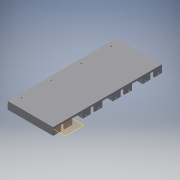
# Autodesk Inventor part: Syring Pump Holder
Saved by Autodesk Inventor 2018.1 (Build 221171000, 171)
## iProperties
Created: 2024-06-08
Part Number: Syring Pump Holder
Material: Generic
Document SubType Name: Modeling
Designer: Enrico
Density: 1 g/cm^3
Appearance: Default
Author: Enrico
Autodesk Inventor part; units mm, degrees
ref_plane "YZ Plane" through (0, 0, 0) normal (1, 0, 0) x (0, 1, 0)
ref_plane "XZ Plane" through (0, 0, 0) normal (0, 1, 0) x (-1, 0, 0)
ref_plane "XY Plane" through (0, 0, 0) normal (0, 0, 1) x (1, 0, 0)
ref_plane "Work Plane1" through (0, 0, 0) normal (0, 0, 1) x (1, 0, 0)
sketch "Sketch1" plane through (0, 0, 0) normal (0, 0, 1) x (1, 0, 0)
  line L0 (57.1, 22.5) -> (57.1, -22.5) construction
  line L1 (57.1, 22.5) -> (-58.1, 22.5) construction
  line L2 (-58.1, 22.5) -> (-58.1, -22.5) construction
  line L3 (-58.1, -22.5) -> (57.1, -22.5) construction
  arc A0 (47.6, -19.5) -> (49.6, -17.5) centre (47.6, -17.5) ccw construction
  line L4 (47.6, -19.5) -> (-47.1, -19.5) construction
  line L5 (-47.1, -19.5) -> (-47.1, -6.5) construction
  arc A1 (-47.1, -6.5) -> (-49.1, -4.5) centre (-49.1, -6.5) ccw construction
  line L6 (-49.1, -4.5) -> (-52.1, -4.5) construction
  arc A2 (-54.1, -2.5) -> (-52.1, -4.5) centre (-52.1, -2.5) ccw construction
  line L7 (-54.1, -2.5) -> (-54.1, 2.5) construction
  arc A3 (-52.1, 4.5) -> (-54.1, 2.5) centre (-52.1, 2.5) ccw construction
  line L8 (-52.1, 4.5) -> (-49.1, 4.5) construction
  arc A4 (-49.1, 4.5) -> (-47.1, 6.5) centre (-49.1, 6.5) ccw construction
  line L9 (-47.1, 6.5) -> (-47.1, 19.5) construction
  line L10 (-47.1, 19.5) -> (47.6, 19.5) construction
  arc A5 (49.6, 17.5) -> (47.6, 19.5) centre (47.6, 17.5) ccw construction
  line L11 (49.6, 17.5) -> (49.6, 9.5) construction
  arc A6 (47.6, 7.5) -> (49.6, 9.5) centre (47.6, 9.5) ccw construction
  line L12 (47.6, 7.5) -> (42.1, 7.5) construction
  arc A7 (42.1, 7.5) -> (40.1, 5.5) centre (42.1, 5.5) ccw construction
  line L13 (40.1, 5.5) -> (40.1, -5.5) construction
  arc A8 (40.1, -5.5) -> (42.1, -7.5) centre (42.1, -5.5) ccw construction
  line L14 (42.1, -7.5) -> (47.6, -7.5) construction
  arc A9 (49.6, -9.5) -> (47.6, -7.5) centre (47.6, -9.5) ccw construction
  line L15 (49.6, -9.5) -> (49.6, -17.5) construction
  line L16 (57.1, 102.5) -> (57.1, 57.5) construction
  line L17 (57.1, 102.5) -> (-58.1, 102.5) construction
  line L18 (-58.1, 102.5) -> (-58.1, 57.5) construction
  line L19 (-58.1, 57.5) -> (57.1, 57.5) construction
  arc A10 (47.6, 60.5) -> (49.6, 62.5) centre (47.6, 62.5) ccw construction
  line L20 (47.6, 60.5) -> (-47.1, 60.5) construction
  line L21 (-47.1, 60.5) -> (-47.1, 73.5) construction
  arc A11 (-47.1, 73.5) -> (-49.1, 75.5) centre (-49.1, 73.5) ccw construction
  line L22 (-49.1, 75.5) -> (-52.1, 75.5) construction
  arc A12 (-54.1, 77.5) -> (-52.1, 75.5) centre (-52.1, 77.5) ccw construction
  line L23 (-54.1, 77.5) -> (-54.1, 82.5) construction
  arc A13 (-52.1, 84.5) -> (-54.1, 82.5) centre (-52.1, 82.5) ccw construction
  line L24 (-52.1, 84.5) -> (-49.1, 84.5) construction
  arc A14 (-49.1, 84.5) -> (-47.1, 86.5) centre (-49.1, 86.5) ccw construction
  line L25 (-47.1, 86.5) -> (-47.1, 99.5) construction
  line L26 (-47.1, 99.5) -> (47.6, 99.5) construction
  arc A15 (49.6, 97.5) -> (47.6, 99.5) centre (47.6, 97.5) ccw construction
  line L27 (49.6, 97.5) -> (49.6, 89.5) construction
  arc A16 (47.6, 87.5) -> (49.6, 89.5) centre (47.6, 89.5) ccw construction
  line L28 (47.6, 87.5) -> (42.1, 87.5) construction
  arc A17 (42.1, 87.5) -> (40.1, 85.5) centre (42.1, 85.5) ccw construction
  line L29 (40.1, 85.5) -> (40.1, 74.5) construction
  arc A18 (40.1, 74.5) -> (42.1, 72.5) centre (42.1, 74.5) ccw construction
  line L30 (42.1, 72.5) -> (47.6, 72.5) construction
  arc A19 (49.6, 70.5) -> (47.6, 72.5) centre (47.6, 70.5) ccw construction
  line L31 (49.6, 70.5) -> (49.6, 62.5) construction
  line L32 (57.1, 182.5) -> (57.1, 137.5) construction
  line L33 (57.1, 182.5) -> (-58.1, 182.5) construction
  line L34 (-58.1, 182.5) -> (-58.1, 137.5) construction
  line L35 (-58.1, 137.5) -> (57.1, 137.5) construction
  arc A20 (47.6, 140.5) -> (49.6, 142.5) centre (47.6, 142.5) ccw construction
  line L36 (47.6, 140.5) -> (-47.1, 140.5) construction
  line L37 (-47.1, 140.5) -> (-47.1, 153.5) construction
  arc A21 (-47.1, 153.5) -> (-49.1, 155.5) centre (-49.1, 153.5) ccw construction
  line L38 (-49.1, 155.5) -> (-52.1, 155.5) construction
  arc A22 (-54.1, 157.5) -> (-52.1, 155.5) centre (-52.1, 157.5) ccw construction
  line L39 (-54.1, 157.5) -> (-54.1, 162.5) construction
  arc A23 (-52.1, 164.5) -> (-54.1, 162.5) centre (-52.1, 162.5) ccw construction
  line L40 (-52.1, 164.5) -> (-49.1, 164.5) construction
  arc A24 (-49.1, 164.5) -> (-47.1, 166.5) centre (-49.1, 166.5) ccw construction
  line L41 (-47.1, 166.5) -> (-47.1, 179.5) construction
  line L42 (-47.1, 179.5) -> (47.6, 179.5) construction
  arc A25 (49.6, 177.5) -> (47.6, 179.5) centre (47.6, 177.5) ccw construction
  line L43 (49.6, 177.5) -> (49.6, 169.5) construction
  arc A26 (47.6, 167.5) -> (49.6, 169.5) centre (47.6, 169.5) ccw construction
  line L44 (47.6, 167.5) -> (42.1, 167.5) construction
  arc A27 (42.1, 167.5) -> (40.1, 165.5) centre (42.1, 165.5) ccw construction
  line L45 (40.1, 165.5) -> (40.1, 154.5) construction
  arc A28 (40.1, 154.5) -> (42.1, 152.5) centre (42.1, 154.5) ccw construction
  line L46 (42.1, 152.5) -> (47.6, 152.5) construction
  arc A29 (49.6, 150.5) -> (47.6, 152.5) centre (47.6, 150.5) ccw construction
  line L47 (49.6, 150.5) -> (49.6, 142.5) construction
  line L48 (57.1, 262.5) -> (57.1, 217.5) construction
  line L49 (57.1, 262.5) -> (-58.1, 262.5) construction
  line L50 (-58.1, 262.5) -> (-58.1, 217.5) construction
  line L51 (-58.1, 217.5) -> (57.1, 217.5) construction
  arc A30 (47.6, 220.5) -> (49.6, 222.5) centre (47.6, 222.5) ccw construction
  line L52 (47.6, 220.5) -> (-47.1, 220.5) construction
  line L53 (-47.1, 220.5) -> (-47.1, 233.5) construction
  arc A31 (-47.1, 233.5) -> (-49.1, 235.5) centre (-49.1, 233.5) ccw construction
  line L54 (-49.1, 235.5) -> (-52.1, 235.5) construction
  arc A32 (-54.1, 237.5) -> (-52.1, 235.5) centre (-52.1, 237.5) ccw construction
  line L55 (-54.1, 237.5) -> (-54.1, 242.5) construction
  arc A33 (-52.1, 244.5) -> (-54.1, 242.5) centre (-52.1, 242.5) ccw construction
  line L56 (-52.1, 244.5) -> (-49.1, 244.5) construction
  arc A34 (-49.1, 244.5) -> (-47.1, 246.5) centre (-49.1, 246.5) ccw construction
  line L57 (-47.1, 246.5) -> (-47.1, 259.5) construction
  line L58 (-47.1, 259.5) -> (47.6, 259.5) construction
  arc A35 (49.6, 257.5) -> (47.6, 259.5) centre (47.6, 257.5) ccw construction
  line L59 (49.6, 257.5) -> (49.6, 249.5) construction
  arc A36 (47.6, 247.5) -> (49.6, 249.5) centre (47.6, 249.5) ccw construction
  line L60 (47.6, 247.5) -> (42.1, 247.5) construction
  arc A37 (42.1, 247.5) -> (40.1, 245.5) centre (42.1, 245.5) ccw construction
  line L61 (40.1, 245.5) -> (40.1, 234.5) construction
  arc A38 (40.1, 234.5) -> (42.1, 232.5) centre (42.1, 234.5) ccw construction
  line L62 (42.1, 232.5) -> (47.6, 232.5) construction
  arc A39 (49.6, 230.5) -> (47.6, 232.5) centre (47.6, 230.5) ccw construction
  line L63 (49.6, 230.5) -> (49.6, 222.5) construction
  circle A40 centre (-49.9, 240) radius 1.5 projected
  arc A41 (-26, 167) -> (-26, 153) centre (-26, 160) ccw construction
  line L64 (-26, 167) -> (26, 167) construction
  arc A42 (26, 153) -> (26, 167) centre (26, 160) ccw construction
  line L65 (26, 153) -> (-26, 153) construction
  circle A43 centre (44.1, 147) radius 1.5 construction
  circle A44 centre (44.1, 173) radius 1.5 construction
  circle A45 centre (-49.9, 160) radius 1.5 projected
  line L66 (47.6, 140.5) -> (-47.1, 140.5) construction
  arc A46 (47.6, 140.5) -> (49.6, 142.5) centre (47.6, 142.5) ccw construction
  line L67 (49.6, 150.5) -> (49.6, 142.5) construction
  arc A47 (49.6, 150.5) -> (47.6, 152.5) centre (47.6, 150.5) ccw construction
  line L68 (42.1, 152.5) -> (47.6, 152.5) construction
  arc A48 (40.1, 154.5) -> (42.1, 152.5) centre (42.1, 154.5) ccw construction
  line L69 (40.1, 165.5) -> (40.1, 154.5) construction
  arc A49 (42.1, 167.5) -> (40.1, 165.5) centre (42.1, 165.5) ccw construction
  line L70 (47.6, 167.5) -> (42.1, 167.5) construction
  arc A50 (47.6, 167.5) -> (49.6, 169.5) centre (47.6, 169.5) ccw construction
  line L71 (49.6, 177.5) -> (49.6, 169.5) construction
  arc A51 (49.6, 177.5) -> (47.6, 179.5) centre (47.6, 177.5) ccw construction
  line L72 (-47.1, 179.5) -> (47.6, 179.5) construction
  line L73 (-47.1, 166.5) -> (-47.1, 179.5) construction
  arc A52 (-49.1, 164.5) -> (-47.1, 166.5) centre (-49.1, 166.5) ccw construction
  line L74 (-52.1, 164.5) -> (-49.1, 164.5) construction
  arc A53 (-52.1, 164.5) -> (-54.1, 162.5) centre (-52.1, 162.5) ccw construction
  line L75 (-54.1, 157.5) -> (-54.1, 162.5) construction
  arc A54 (-54.1, 157.5) -> (-52.1, 155.5) centre (-52.1, 157.5) ccw construction
  line L76 (-49.1, 155.5) -> (-52.1, 155.5) construction
  arc A55 (-47.1, 153.5) -> (-49.1, 155.5) centre (-49.1, 153.5) ccw construction
  line L77 (-47.1, 140.5) -> (-47.1, 153.5) construction
  arc A56 (-26, 87) -> (-26, 73) centre (-26, 80) ccw construction
  line L78 (-26, 87) -> (26, 87) construction
  arc A57 (26, 73) -> (26, 87) centre (26, 80) ccw construction
  line L79 (26, 73) -> (-26, 73) construction
  circle A58 centre (44.1, 67) radius 1.5 construction
  circle A59 centre (44.1, 93) radius 1.5 construction
  circle A60 centre (-49.9, 80) radius 1.5 projected
  line L80 (47.6, 60.5) -> (-47.1, 60.5) construction
  arc A61 (47.6, 60.5) -> (49.6, 62.5) centre (47.6, 62.5) ccw construction
  line L81 (49.6, 70.5) -> (49.6, 62.5) construction
  arc A62 (49.6, 70.5) -> (47.6, 72.5) centre (47.6, 70.5) ccw construction
  line L82 (42.1, 72.5) -> (47.6, 72.5) construction
  arc A63 (40.1, 74.5) -> (42.1, 72.5) centre (42.1, 74.5) ccw construction
  line L83 (40.1, 85.5) -> (40.1, 74.5) construction
  arc A64 (42.1, 87.5) -> (40.1, 85.5) centre (42.1, 85.5) ccw construction
  line L84 (47.6, 87.5) -> (42.1, 87.5) construction
  arc A65 (47.6, 87.5) -> (49.6, 89.5) centre (47.6, 89.5) ccw construction
  line L85 (49.6, 97.5) -> (49.6, 89.5) construction
  arc A66 (49.6, 97.5) -> (47.6, 99.5) centre (47.6, 97.5) ccw construction
  line L86 (-47.1, 99.5) -> (47.6, 99.5) construction
  line L87 (-47.1, 86.5) -> (-47.1, 99.5) construction
  arc A67 (-49.1, 84.5) -> (-47.1, 86.5) centre (-49.1, 86.5) ccw construction
  line L88 (-52.1, 84.5) -> (-49.1, 84.5) construction
  arc A68 (-52.1, 84.5) -> (-54.1, 82.5) centre (-52.1, 82.5) ccw construction
  line L89 (-54.1, 77.5) -> (-54.1, 82.5) construction
  arc A69 (-54.1, 77.5) -> (-52.1, 75.5) centre (-52.1, 77.5) ccw construction
  line L90 (-49.1, 75.5) -> (-52.1, 75.5) construction
  arc A70 (-47.1, 73.5) -> (-49.1, 75.5) centre (-49.1, 73.5) ccw construction
  line L91 (-47.1, 60.5) -> (-47.1, 73.5) construction
  arc A71 (-26, 7) -> (-26, -7) centre (-26, 0) ccw construction
  line L92 (-26, 7) -> (26, 7) construction
  arc A72 (26, -7) -> (26, 7) centre (26, 0) ccw construction
  line L93 (26, -7) -> (-26, -7) construction
  circle A73 centre (44.1, -13) radius 1.5 construction
  circle A74 centre (44.1, 13) radius 1.5 construction
  circle A75 centre (-49.9, 0) radius 1.5 projected
  line L94 (47.6, -19.5) -> (-47.1, -19.5) construction
  arc A76 (47.6, -19.5) -> (49.6, -17.5) centre (47.6, -17.5) ccw construction
  line L95 (49.6, -9.5) -> (49.6, -17.5) construction
  arc A77 (49.6, -9.5) -> (47.6, -7.5) centre (47.6, -9.5) ccw construction
  line L96 (42.1, -7.5) -> (47.6, -7.5) construction
  arc A78 (40.1, -5.5) -> (42.1, -7.5) centre (42.1, -5.5) ccw construction
  line L97 (40.1, 5.5) -> (40.1, -5.5) construction
  arc A79 (42.1, 7.5) -> (40.1, 5.5) centre (42.1, 5.5) ccw construction
  line L98 (47.6, 7.5) -> (42.1, 7.5) construction
  arc A80 (47.6, 7.5) -> (49.6, 9.5) centre (47.6, 9.5) ccw construction
  line L99 (49.6, 17.5) -> (49.6, 9.5) construction
  arc A81 (49.6, 17.5) -> (47.6, 19.5) centre (47.6, 17.5) ccw construction
  line L100 (-47.1, 19.5) -> (47.6, 19.5) construction
  line L101 (-47.1, 6.5) -> (-47.1, 19.5) construction
  arc A82 (-49.1, 4.5) -> (-47.1, 6.5) centre (-49.1, 6.5) ccw construction
  line L102 (-52.1, 4.5) -> (-49.1, 4.5) construction
  arc A83 (-52.1, 4.5) -> (-54.1, 2.5) centre (-52.1, 2.5) ccw construction
  line L103 (-54.1, -2.5) -> (-54.1, 2.5) construction
  arc A84 (-54.1, -2.5) -> (-52.1, -4.5) centre (-52.1, -2.5) ccw construction
  line L104 (-49.1, -4.5) -> (-52.1, -4.5) construction
  arc A85 (-47.1, -6.5) -> (-49.1, -4.5) centre (-49.1, -6.5) ccw construction
  line L105 (-47.1, -19.5) -> (-47.1, -6.5) construction
  arc A86 (-26, 247) -> (-26, 233) centre (-26, 240) ccw construction
  line L106 (-26, 247) -> (26, 247) construction
  arc A87 (26, 233) -> (26, 247) centre (26, 240) ccw construction
  line L107 (26, 233) -> (-26, 233) construction
  circle A88 centre (44.1, 227) radius 1.5 construction
  circle A89 centre (44.1, 253) radius 1.5 construction
  circle A90 centre (-49.9, 240) radius 1.5 construction
  line L108 (47.6, 220.5) -> (-47.1, 220.5) construction
  arc A91 (47.6, 220.5) -> (49.6, 222.5) centre (47.6, 222.5) ccw construction
  line L109 (49.6, 230.5) -> (49.6, 222.5) construction
  arc A92 (49.6, 230.5) -> (47.6, 232.5) centre (47.6, 230.5) ccw construction
  line L110 (42.1, 232.5) -> (47.6, 232.5) construction
  arc A93 (40.1, 234.5) -> (42.1, 232.5) centre (42.1, 234.5) ccw construction
  line L111 (40.1, 245.5) -> (40.1, 234.5) construction
  arc A94 (42.1, 247.5) -> (40.1, 245.5) centre (42.1, 245.5) ccw construction
  line L112 (47.6, 247.5) -> (42.1, 247.5) construction
  arc A95 (47.6, 247.5) -> (49.6, 249.5) centre (47.6, 249.5) ccw construction
  line L113 (49.6, 257.5) -> (49.6, 249.5) construction
  arc A96 (49.6, 257.5) -> (47.6, 259.5) centre (47.6, 257.5) ccw construction
  line L114 (-47.1, 259.5) -> (47.6, 259.5) construction
  line L115 (-47.1, 246.5) -> (-47.1, 259.5) construction
  arc A97 (-49.1, 244.5) -> (-47.1, 246.5) centre (-49.1, 246.5) ccw construction
  line L116 (-52.1, 244.5) -> (-49.1, 244.5) construction
  arc A98 (-52.1, 244.5) -> (-54.1, 242.5) centre (-52.1, 242.5) ccw construction
  line L117 (-54.1, 237.5) -> (-54.1, 242.5) construction
  arc A99 (-54.1, 237.5) -> (-52.1, 235.5) centre (-52.1, 237.5) ccw construction
  line L118 (-49.1, 235.5) -> (-52.1, 235.5) construction
  arc A100 (-47.1, 233.5) -> (-49.1, 235.5) centre (-49.1, 233.5) ccw construction
  line L119 (-47.1, 220.5) -> (-47.1, 233.5) construction
  line L120 (60.4, 265.8) -> (-61.4, 265.8)
  line L121 (-61.4, 265.8) -> (-61.4, -25.8)
  line L122 (-61.4, -25.8) -> (60.4, -25.8)
  line L123 (60.4, -25.8) -> (60.4, 265.8)
  point P0 (0, 0)
  dimension "d0" = 3.3
  dimension "d1" = 3.3
  dimension "d2" = 3.3
  dimension "d3" = 3.3
  constraints: 8 end point, 2 parallel, 1 horizontal, 1 perpendicular
  measures "d0" distance between parallel lines of L49 L120
  measures "d1" distance between parallel lines of L48 L123
  measures "d2" distance between parallel lines of L50 L121
  measures "d3" distance between parallel lines of L3 L122
extrude "Extrusion1" add sketch "Sketch1" along normal blind 5
sketch "Sketch2" plane through (0, 0, 0) normal (0, 0, -1) x (-1, 0, 0)
  line L0 (-57.1, -22.5) -> (-57.1, 22.5) construction
  line L1 (-57.1, -22.5) -> (58.1, -22.5) construction
  line L2 (58.1, -22.5) -> (58.1, 22.5) construction
  line L3 (58.1, 22.5) -> (-57.1, 22.5) construction
  circle A0 centre (-55.1, -16.5) radius 1.5 construction
  circle A1 centre (-55.1, 16.5) radius 1.5 construction
  line L4 (-57.1, 57.5) -> (-57.1, 102.5) construction
  line L5 (-57.1, 57.5) -> (58.1, 57.5) construction
  line L6 (58.1, 57.5) -> (58.1, 102.5) construction
  line L7 (58.1, 102.5) -> (-57.1, 102.5) construction
  circle A2 centre (-55.1, 63.5) radius 1.5 construction
  circle A3 centre (-55.1, 96.5) radius 1.5 construction
  line L8 (-57.1, 137.5) -> (-57.1, 182.5) construction
  line L9 (-57.1, 137.5) -> (58.1, 137.5) construction
  line L10 (58.1, 137.5) -> (58.1, 182.5) construction
  line L11 (58.1, 182.5) -> (-57.1, 182.5) construction
  circle A4 centre (-55.1, 143.5) radius 1.5 construction
  circle A5 centre (-55.1, 176.5) radius 1.5 construction
  line L12 (-57.1, 217.5) -> (-57.1, 262.5) construction
  line L13 (-57.1, 217.5) -> (58.1, 217.5) construction
  line L14 (58.1, 217.5) -> (58.1, 262.5) construction
  line L15 (58.1, 262.5) -> (-57.1, 262.5) construction
  circle A6 centre (-55.1, 223.5) radius 1.5 construction
  circle A7 centre (-55.1, 256.5) radius 1.5 construction
  line L16 (58.4, 217.2) -> (-57.4, 217.2)
  line L17 (-57.4, 217.2) -> (-57.4, 262.8)
  line L18 (-57.4, 262.8) -> (58.4, 262.8)
  line L19 (58.4, 262.8) -> (58.4, 217.2)
  line L20 (58.4, 137.2) -> (-57.4, 137.2)
  line L21 (-57.4, 137.2) -> (-57.4, 182.8)
  line L22 (-57.4, 182.8) -> (58.4, 182.8)
  line L23 (58.4, 182.8) -> (58.4, 137.2)
  line L24 (58.4, 57.2) -> (-57.4, 57.2)
  line L25 (-57.4, 57.2) -> (-57.4, 102.8)
  line L26 (-57.4, 102.8) -> (58.4, 102.8)
  line L27 (58.4, 102.8) -> (58.4, 57.2)
  line L28 (58.4, -22.8) -> (-57.4, -22.8)
  line L29 (-57.4, -22.8) -> (-57.4, 22.8)
  line L30 (-57.4, 22.8) -> (58.4, 22.8)
  line L31 (58.4, 22.8) -> (58.4, -22.8)
  line L32 (-60.4, -25.8) -> (61.4, -25.8)
  line L33 (61.4, -25.8) -> (61.4, 25.8)
  line L34 (61.4, 25.8) -> (-60.4, 25.8)
  line L35 (-60.4, 25.8) -> (-60.4, -25.8)
  line L36 (-60.4, 54.2) -> (61.4, 54.2)
  line L37 (61.4, 54.2) -> (61.4, 105.8)
  line L38 (61.4, 105.8) -> (-60.4, 105.8)
  line L39 (-60.4, 105.8) -> (-60.4, 54.2)
  line L40 (-60.4, 134.2) -> (61.4, 134.2)
  line L41 (61.4, 134.2) -> (61.4, 185.8)
  line L42 (61.4, 185.8) -> (-60.4, 185.8)
  line L43 (-60.4, 185.8) -> (-60.4, 134.2)
  line L44 (-60.4, 214.2) -> (61.4, 214.2)
  line L45 (61.4, 214.2) -> (61.4, 265.8)
  line L46 (61.4, 265.8) -> (-60.4, 265.8)
  line L47 (-60.4, 265.8) -> (-60.4, 214.2)
  line L48 (-85.2, 244.5) -> (-85.2, 235.5) projected
  line L49 (-58.1, 244.5) -> (-85.2, 244.5) projected
  line L50 (-58.1, 235.5) -> (-58.1, 244.5) projected
  line L51 (-85.2, 235.5) -> (-58.1, 235.5) projected
  line L52 (-85.2, 164.5) -> (-85.2, 155.5) projected
  line L53 (-58.1, 164.5) -> (-85.2, 164.5) projected
  line L54 (-58.1, 155.5) -> (-58.1, 164.5) projected
  line L55 (-85.2, 155.5) -> (-58.1, 155.5) projected
  line L56 (-85.2, 84.5) -> (-85.2, 75.5) projected
  line L57 (-58.1, 84.5) -> (-85.2, 84.5) projected
  line L58 (-58.1, 75.5) -> (-58.1, 84.5) projected
  line L59 (-85.2, 75.5) -> (-58.1, 75.5) projected
  line L60 (-85.2, 4.5) -> (-85.2, -4.5) projected
  line L61 (-58.1, 4.5) -> (-85.2, 4.5) projected
  line L62 (-58.1, -4.5) -> (-58.1, 4.5) projected
  line L63 (-85.2, -4.5) -> (-58.1, -4.5) projected
  line L64 (-85.5, 244.8) -> (-85.5, 235.2)
  line L65 (-85.5, 235.2) -> (-57.8, 235.2)
  line L66 (-57.8, 235.2) -> (-57.8, 244.8)
  line L67 (-57.8, 244.8) -> (-85.5, 244.8)
  line L68 (-85.5, 164.8) -> (-85.5, 155.2)
  line L69 (-85.5, 155.2) -> (-57.8, 155.2)
  line L70 (-57.8, 155.2) -> (-57.8, 164.8)
  line L71 (-57.8, 164.8) -> (-85.5, 164.8)
  line L72 (-85.5, 84.8) -> (-85.5, 75.2)
  line L73 (-85.5, 75.2) -> (-57.8, 75.2)
  line L74 (-57.8, 75.2) -> (-57.8, 84.8)
  line L75 (-57.8, 84.8) -> (-85.5, 84.8)
  line L76 (-85.5, 4.8) -> (-85.5, -4.8)
  line L77 (-85.5, -4.8) -> (-57.8, -4.8)
  line L78 (-57.8, -4.8) -> (-57.8, 4.8)
  line L79 (-57.8, 4.8) -> (-85.5, 4.8) construction
  line L80 (-57.4, 4.8) -> (-60.4, 4.8)
  line L81 (-57.4, -4.8) -> (-60.4, -4.8)
  line L82 (-57.4, 84.8) -> (-60.4, 84.8)
  line L83 (-57.4, 75.2) -> (-60.4, 75.2)
  line L84 (-57.4, 164.8) -> (-60.4, 164.8)
  line L85 (-57.4, 155.2) -> (-60.4, 155.2)
  line L86 (-57.4, 244.8) -> (-60.4, 244.8)
  line L87 (-57.4, 235.2) -> (-60.4, 235.2)
  line L88 (-57.4, 244.8) -> (-60.4, 244.8)
  line L89 (-60.4, 244.8) -> (-60.4, 235.2)
  line L90 (-60.4, 235.2) -> (-57.4, 235.2)
  line L91 (-57.4, 235.2) -> (-57.4, 244.8)
  line L92 (-57.4, 164.8) -> (-60.4, 164.8)
  line L93 (-60.4, 164.8) -> (-60.4, 155.2)
  line L94 (-60.4, 155.2) -> (-57.4, 155.2)
  line L95 (-57.4, 155.2) -> (-57.4, 164.8)
  line L96 (-57.4, 84.8) -> (-60.4, 84.8)
  line L97 (-60.4, 84.8) -> (-60.4, 75.2)
  line L98 (-60.4, 75.2) -> (-57.4, 75.2)
  line L99 (-57.4, 75.2) -> (-57.4, 84.8)
  point P0 (0, 0)
  dimension "d6" = 0.3
  dimension "d7" = 0.3
  dimension "d8" = 0.3
  dimension "d9" = 0.3
  dimension "d10" = 3
  dimension "d11" = 3
  dimension "d12" = 3
  dimension "d13" = 3
  dimension "d14" = 0.3
  dimension "d15" = 0.3
  dimension "d16" = 0.3
  dimension "d17" = 0.3
  dimension "d20" = 80
  constraints: 136 end point, 6 parallel, 6 point on line, 3 horizontal, 3 perpendicular, 2 collinear, 1 vertical, 54 other
  measures "d6" distance between parallel lines of L13 L16
  measures "d7" distance between parallel lines of L9 L20
  measures "d8" distance between parallel lines of L5 L24
  measures "d9" distance between parallel lines of L1 L28
  measures "d10" distance between parallel lines of L28 L32
  measures "d11" distance between parallel lines of L24 L36
  measures "d12" distance between parallel lines of L20 L40
  measures "d13" distance between parallel lines of L16 L44
  measures "d14" distance between parallel lines of L49 L67
  measures "d15" distance between parallel lines of L53 L71
  measures "d16" distance between parallel lines of L57 L75
  measures "d17" distance between parallel lines of L61 L79
  measures "d20" distance of L80.start L82.start
extrude "Extrusion2" add sketch "Sketch2" along normal blind 15 contours L19 L18 L17 L86 L67 L47 L46 L45 L44 L65 L87 L16 | L23 L22 L21 L84 L71 L43 L42 L41 L40 L69 L85 L20 | L27 L26 L25 L82 L75 L39 L38 L37 L36 L73 L83 L24 | L31 L30 L29 L80 L35 L34 L33 L32 L77 L81 L28
sketch "Sketch3" plane through (60.4, -25.8, 5) normal (1, 0, 0) x (0, 0, -1)
  circle A0 centre (16.1, 8.55) radius 1.5 construction
  circle A1 centre (86.1, 43.05) radius 1.5 construction
  circle A2 centre (16.1, 43.05) radius 1.5 construction
  circle A3 centre (86.1, 8.55) radius 1.5 construction
  line L0 (6.1, 30.3) -> (44.6, 30.3) construction
  line L1 (44.6, 30.3) -> (44.6, 21.3) construction
  line L2 (44.6, 21.3) -> (6.1, 21.3) construction
  line L3 (6.1, 4.3) -> (6.1, 21.3) construction
  line L4 (131.1, 4.3) -> (6.1, 4.3) construction
  line L5 (131.1, 25.8) -> (131.1, 4.3) construction
  circle A4 centre (111.6, 25.8) radius 19.5 construction
  line L6 (131.1, 47.3) -> (131.1, 25.8) construction
  line L7 (6.1, 47.3) -> (131.1, 47.3) construction
  line L8 (6.1, 30.3) -> (6.1, 47.3) construction
  circle A5 centre (16.1, 88.55) radius 1.5 construction
  circle A6 centre (86.1, 123.05) radius 1.5 construction
  circle A7 centre (16.1, 123.05) radius 1.5 construction
  circle A8 centre (86.1, 88.55) radius 1.5 construction
  line L9 (6.1, 110.3) -> (44.6, 110.3) construction
  line L10 (44.6, 110.3) -> (44.6, 101.3) construction
  line L11 (44.6, 101.3) -> (6.1, 101.3) construction
  line L12 (6.1, 84.3) -> (6.1, 101.3) construction
  line L13 (131.1, 84.3) -> (6.1, 84.3) construction
  line L14 (131.1, 105.8) -> (131.1, 84.3) construction
  circle A9 centre (111.6, 105.8) radius 19.5 construction
  line L15 (131.1, 127.3) -> (131.1, 105.8) construction
  line L16 (6.1, 127.3) -> (131.1, 127.3) construction
  line L17 (6.1, 110.3) -> (6.1, 127.3) construction
  circle A10 centre (16.1, 168.55) radius 1.5 construction
  circle A11 centre (86.1, 203.05) radius 1.5 construction
  circle A12 centre (16.1, 203.05) radius 1.5 construction
  circle A13 centre (86.1, 168.55) radius 1.5 construction
  line L18 (6.1, 190.3) -> (44.6, 190.3) construction
  line L19 (44.6, 190.3) -> (44.6, 181.3) construction
  line L20 (44.6, 181.3) -> (6.1, 181.3) construction
  line L21 (6.1, 164.3) -> (6.1, 181.3) construction
  line L22 (131.1, 164.3) -> (6.1, 164.3) construction
  line L23 (131.1, 185.8) -> (131.1, 164.3) construction
  circle A14 centre (111.6, 185.8) radius 19.5 construction
  line L24 (131.1, 207.3) -> (131.1, 185.8) construction
  line L25 (6.1, 207.3) -> (131.1, 207.3) construction
  line L26 (6.1, 190.3) -> (6.1, 207.3) construction
  circle A15 centre (16.1, 248.55) radius 1.5 construction
  circle A16 centre (86.1, 283.05) radius 1.5 construction
  circle A17 centre (16.1, 283.05) radius 1.5 construction
  circle A18 centre (86.1, 248.55) radius 1.5 construction
  line L27 (6.1, 270.3) -> (44.6, 270.3) construction
  line L28 (44.6, 270.3) -> (44.6, 261.3) construction
  line L29 (44.6, 261.3) -> (6.1, 261.3) construction
  line L30 (6.1, 244.3) -> (6.1, 261.3) construction
  line L31 (131.1, 244.3) -> (6.1, 244.3) construction
  line L32 (131.1, 265.8) -> (131.1, 244.3) construction
  circle A19 centre (111.6, 265.8) radius 19.5 construction
  line L33 (131.1, 287.3) -> (131.1, 265.8) construction
  line L34 (6.1, 287.3) -> (131.1, 287.3) construction
  line L35 (6.1, 270.3) -> (6.1, 287.3) construction
  circle A20 centre (16.1, 8.55) radius 1.8
  circle A21 centre (16.1, 43.05) radius 1.8
  circle A22 centre (16.1, 88.55) radius 1.8
  circle A23 centre (16.1, 123.05) radius 1.8
  circle A24 centre (16.1, 168.55) radius 1.8
  circle A25 centre (16.1, 203.05) radius 1.8
  circle A26 centre (16.1, 248.55) radius 1.8
  circle A27 centre (16.1, 283.05) radius 1.8
  point P0 (5, 25.8)
  dimension "d27" = 0.3
  dimension "d28" = 0.3
  dimension "d29" = 0.3
  dimension "d30" = 0.3
  dimension "d31" = 0.3
  dimension "d32" = 0.3
  dimension "d33" = 0.3
  dimension "d34" = 0.3
  constraints: 8 centre point, 4 horizontal alignment
  measures "d27" radial gap between concentric circles of A0 A20
  measures "d28" radial gap between concentric circles of A2 A21
  measures "d29" radial gap between concentric circles of A5 A22
  measures "d30" radial gap between concentric circles of A7 A23
  measures "d31" radial gap between concentric circles of A10 A24
  measures "d32" radial gap between concentric circles of A12 A25
  measures "d33" radial gap between concentric circles of A15 A26
  measures "d34" radial gap between concentric circles of A17 A27
extrude "Extrusion3" cut sketch "Sketch3" against normal up to next
ref_plane "Work Plane2" through (-61.4, 120, 5) normal (0, 1, 0) x (1, 0, 0)
sketch "Sketch4" plane through (0, 0, 0) normal (0, 0, -1) x (-1, 0, 0)
  circle A0 centre (46.4, 200) radius 3.15
  circle A1 centre (-45.4, 200) radius 3.15
  line L0 (61.4, 214.2) -> (61.4, 185.8) projected
  line L1 (-60.4, 185.8) -> (-60.4, 214.2) projected
  line L2 (61.4, 265.8) -> (61.4, -25.8) projected
  line L3 (61.4, 120) -> (-60.4, 120) construction
  circle A2 centre (46.4, 40) radius 3.15
  circle A3 centre (-45.4, 40) radius 3.15
  point P0 (0, 0)
  point P1 (61.4, 200)
  dimension "d37" = 6.3
  dimension "d38" = 6.3
  dimension "d41" = 15
  dimension "d42" = 15
  constraints: 4 centre point, 2 end point, 2 horizontal alignment, 2 midpoint, 2 symmetric about line, 1 horizontal, 2 other
  measures "d37" diameter of A0
  measures "d38" diameter of A1
  measures "d41" distance from line of L0 A0.centre
  measures "d42" distance from line of L1 A1.centre
extrude "Extrusion4" cut sketch "Sketch4" against normal up to next
sketch "Sketch5" plane through (0, 0, 5) normal (0, 0, 1) x (1, 0, 0)
  line L0 (157.7, -40.393) -> (-71.4, -40.393)
  line L1 (-71.4, -40.393) -> (-71.4, 280.393)
  line L2 (-71.4, 280.393) -> (157.7, 280.393)
  line L3 (157.7, 280.393) -> (157.7, -40.393)
  arc A0 (146.924, 34.8766) -> (146.924, 45.1234) centre (130.4, 40) ccw projected
  line L4 (84.2088, -23.322) -> (91.2798, -30.393)
  line L5 (84.2088, 263.322) -> (91.2798, 270.393)
  line L6 (-61.4, 265.8) -> (-61.4, -25.8) projected
  point P0 (0, 0)
  point P1 (147.7, 40)
  dimension "d45" = 10
  dimension "d46" = 10
  dimension "d47" = 10
  dimension "d48" = 10
  dimension "d49" = 320.7861
  dimension "d50" = 229.1
  constraints: 12 end point, 2 parallel, 1 horizontal, 1 perpendicular, 1 point on circle, 6 other
  measures "d45" distance from line of L4.end L0
  measures "d46" distance from line of L5.end L2
  measures "d47" distance between parallel lines of L6 L1
  measures "d48" distance from line of point (147.7, 40) L3
  measures "d49" distance of L0.end L1.end
  measures "d50" distance of L0.start L0.end
body "Solid1"
